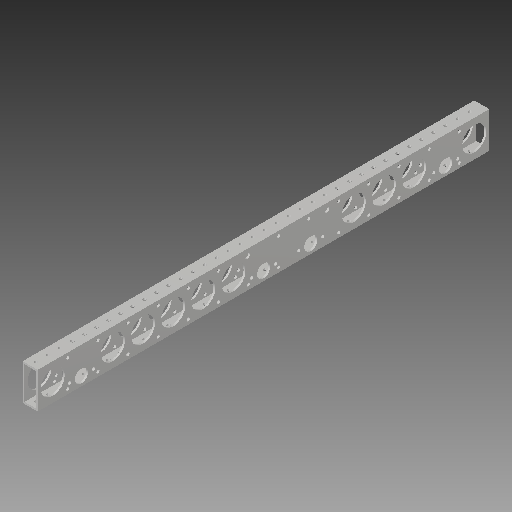
# Autodesk Inventor part: Side Extrusion
Saved by Autodesk Inventor 2019.4 (Build 234330000, 330)
## iProperties
Created: 2019-12-11
Part Number: Side Extrusion
Material: Aluminum 6061
Document SubType Name: Modeling
Designer: Mark
Mass: 702.477 g
Surface Area: 1912.79 cm^2
Volume: 260.177 cm^3
Density: 2.7 g/cm^3
Appearance: Aluminum - Flat
Author: Mark
Autodesk Inventor part; units mm, degrees
ref_plane "YZ Plane" through (0, 0, 0) normal (1, 0, 0) x (0, 1, 0)
ref_plane "XZ Plane" through (0, 0, 0) normal (0, 1, 0) x (-1, 0, 0)
ref_plane "XY Plane" through (0, 0, 0) normal (0, 0, 1) x (1, 0, 0)
sketch "Sketch1" plane through (0, 0, 0) normal (0, 0, 1) x (1, 0, 0)
  line L0 (-12.5, -30) -> (12.5, -30)
  line L1 (12.5, -30) -> (12.5, 30)
  line L2 (12.5, 30) -> (-12.5, 30)
  line L3 (-12.5, 30) -> (-12.5, -30)
  line L4 (-12.5, -30) -> (12.5, 30) construction
  line L5 (12.5, -30) -> (-12.5, 30) construction
  line L6 (-9.5, -27) -> (9.5, -27)
  line L7 (9.5, -27) -> (9.5, 27)
  line L8 (9.5, 27) -> (-9.5, 27)
  line L9 (-9.5, 27) -> (-9.5, -27)
  line L10 (-9.5, -27) -> (9.5, 27) construction
  line L11 (9.5, -27) -> (-9.5, 27) construction
  point P0 (0, 0)
  dimension "d0" = 25
  dimension "d1" = 60
  dimension "d2" = 19
  dimension "d3" = 54
  constraints: 24 end point, 4 midpoint, 4 parallel, 2 horizontal, 2 perpendicular
  measures "d0" distance of L2.end L1.end
  measures "d1" distance of L1.end L0.end
  measures "d2" distance of L8.end L7.end
  measures "d3" distance of L7.end L6.end
extrude "Extrusion1" add sketch "Sketch1" along normal blind 750
sketch "Sketch2" plane through (12.5, -30, 0) normal (1, 0, 0) x (0, 0, -1)
  circle A0 centre (-375, 15) radius 11
  circle A1 centre (-677.46, 15) radius 11
  circle A2 centre (-72.54, 15) radius 11
  line L0 (0, 60) -> (-750, 60) projected
  line L1 (-750, 0) -> (-750, 60) projected
  circle A3 centre (-677.46, 15) radius 20 construction
  circle A4 centre (-697.46, 15) radius 2.75
  circle A5 centre (-657.46, 15) radius 2.75
  line L2 (-677.46, 15) -> (-697.46, 15) construction
  line L3 (-677.46, 15) -> (-657.46, 15) construction
  line L4 (-375, 15) -> (-375, 60)
  circle A6 centre (-395, 15) radius 2.75
  line L5 (0, 0) -> (-750, 0) projected
  circle A7 centre (-52.54, 15) radius 2.75
  circle A8 centre (-92.54, 15) radius 2.75
  circle A9 centre (-355, 15) radius 2.75
  circle A10 centre (-316.54, 15) radius 2.75
  circle A11 centre (-276.54, 15) radius 2.75
  circle A12 centre (-296.54, 15) radius 11
  point P0 (0, 30)
  dimension "d6" = 22
  dimension "d7" = 22
  dimension "d8" = 22
  dimension "d9" = 45
  dimension "d10" = 45
  dimension "d11" = 45
  dimension "d12" = 375
  dimension "d13" = 302.46
  dimension "d14" = 302.46
  dimension "d33" = 40
  dimension "d34" = 5.5
  dimension "d35" = 5.5
  dimension "d36" = 40
  dimension "d37" = 180
  dimension "d38" = 5.5
  dimension "d39" = 20
  dimension "d41" = 45
  dimension "d44" = 78.46
  constraints: 13 centre point, 6 end point, 3 horizontal, 3 symmetric about line, 2 point on circle, 1 coincident, 1 collinear, 1 midpoint, 9 other
  measures "d6" diameter of A0
  measures "d7" diameter of A1
  measures "d8" diameter of A2
  measures "d9" distance from line of L0 L4.start
  measures "d10" distance from line of L0 A2.centre
  measures "d11" distance from line of L0 A1.centre
  measures "d12" distance from line of L1 L4.start
  measures "d13" distance of L4.start A1.centre
  measures "d14" distance of L4.start A2.centre
  measures "d33" diameter of A3
  measures "d34" diameter of A4
  measures "d35" diameter of A5
  measures "d36" distance of A5.centre L2.end
  measures "d37" angle of L2 L3
  measures "d38" diameter of A6
  measures "d39" distance of L4.start A6.centre
  measures "d41" distance from line of L0 A6.centre
  measures "d44" distance of A6.centre A10.centre
extrude "Extrusion2" cut sketch "Sketch2" against normal through all
sketch "Sketch4" plane through (-12.5, 30, 0) normal (0, 1, 0) x (1, 0, 0)
  circle A0 centre (12.5, -20) radius 2.75
  line L0 (25, 0) -> (25, -750) projected
  line L1 (25, 0) -> (0, 0) projected
  circle A1 centre (12.5, -40) radius 2.75
  circle A2 centre (12.5, -60) radius 2.75
  circle A3 centre (12.5, -80) radius 2.75
  circle A4 centre (12.5, -100) radius 2.75
  circle A5 centre (12.5, -120) radius 2.75
  circle A6 centre (12.5, -140) radius 2.75
  circle A7 centre (12.5, -160) radius 2.75
  circle A8 centre (12.5, -180) radius 2.75
  circle A9 centre (12.5, -200) radius 2.75
  circle A10 centre (12.5, -220) radius 2.75
  circle A11 centre (12.5, -240) radius 2.75
  circle A12 centre (12.5, -260) radius 2.75
  circle A13 centre (12.5, -280) radius 2.75
  circle A14 centre (12.5, -300) radius 2.75
  circle A15 centre (12.5, -320) radius 2.75
  circle A16 centre (12.5, -340) radius 2.75
  circle A17 centre (12.5, -360) radius 2.75
  circle A18 centre (12.5, -380) radius 2.75
  circle A19 centre (12.5, -400) radius 2.75
  circle A20 centre (12.5, -420) radius 2.75
  circle A21 centre (12.5, -440) radius 2.75
  circle A22 centre (12.5, -460) radius 2.75
  circle A23 centre (12.5, -480) radius 2.75
  circle A24 centre (12.5, -500) radius 2.75
  circle A25 centre (12.5, -520) radius 2.75
  circle A26 centre (12.5, -540) radius 2.75
  circle A27 centre (12.5, -560) radius 2.75
  circle A28 centre (12.5, -580) radius 2.75
  circle A29 centre (12.5, -600) radius 2.75
  circle A30 centre (12.5, -620) radius 2.75
  circle A31 centre (12.5, -640) radius 2.75
  circle A32 centre (12.5, -660) radius 2.75
  circle A33 centre (12.5, -680) radius 2.75
  circle A34 centre (12.5, -700) radius 2.75
  circle A35 centre (12.5, -720) radius 2.75
  circle A36 centre (12.5, -740) radius 2.75
  circle A37 centre (12.5, -760) radius 2.75
  circle A38 centre (12.5, -780) radius 2.75
  circle A39 centre (12.5, -800) radius 2.75
  point P0 (12.5, 0)
  dimension "d21" = 5.5
  dimension "d22" = 12.5
  dimension "d23" = 20
  dimension "d26" = 20
  constraints: 40 centre point, 1 vertical, 78 other
  measures "d21" diameter of A0
  measures "d22" distance from line of L0 A0.centre
  measures "d23" distance from line of L1 A0.centre
  measures "d26" distance of A0.centre A1.centre
extrude "Extrusion3" cut sketch "Sketch4" against normal blind 100 contours A0 | A1 | A2 | A3 | A4 | A5 | A6 | A7 | A8 | A9 | A10 | A11 | A12 | A13 | A14 | A15 | A16 | A17 | A18 | A19 | A20 | A21 | A22 | A23 | A24 | A25 | A26 | A27 | A28 | A29 | A30 | A31 | A32 | A33 | A34 | A35 | A36 | A37 | A38
sketch "Sketch5" plane through (12.5, -30, 0) normal (1, 0, 0) x (0, 0, -1)
  circle A0 centre (-401.79, 50) radius 4.25
  line L0 (0, 60) -> (-750, 60) projected
  line L1 (-750, 0) -> (-750, 60) projected
  circle A1 centre (-269.75, 50) radius 4.25
  point P0 (0, 30)
  dimension "d49" = 8.5
  dimension "d50" = 10
  dimension "d51" = 348.21
  dimension "d52" = 8.5
  dimension "d53" = 10
  dimension "d54" = 132.04
  constraints: 2 centre point
  measures "d49" diameter of A0
  measures "d50" distance from line of L0 A0.centre
  measures "d51" distance from line of L1 A0.centre
  measures "d52" diameter of A1
  measures "d53" distance from line of L0 A1.centre
  measures "d54" distance of A0.centre A1.centre
extrude "Extrusion4" cut sketch "Sketch5" against normal blind 50
sketch "Sketch6" plane through (12.5, -30, 0) normal (1, 0, 0) x (0, 0, -1)
  line L0 (0, 60) -> (-750, 60) projected
  line L1 (-375, 60) -> (-375, 0) construction
  line L2 (-375, 60) -> (-315, 60) construction
  circle A0 centre (-375, 30) radius 20
  line L3 (-400, 7.5) -> (-350, 7.5) construction
  line L4 (-350, 7.5) -> (-350, 52.5) construction
  line L5 (-350, 52.5) -> (-400, 52.5) construction
  line L6 (-400, 52.5) -> (-400, 7.5) construction
  line L7 (-400, 7.5) -> (-350, 52.5) construction
  line L8 (-350, 7.5) -> (-400, 52.5) construction
  circle A1 centre (-350, 52.5) radius 2.75
  circle A2 centre (-400, 52.5) radius 2.75
  circle A3 centre (-400, 7.5) radius 2.75
  circle A4 centre (-350, 7.5) radius 2.75
  circle A5 centre (-450, 52.5) radius 2.75
  circle A6 centre (-450, 7.5) radius 2.75
  circle A7 centre (-400, 7.5) radius 2.75
  circle A8 centre (-425, 30) radius 20
  circle A9 centre (-400, 52.5) radius 2.75
  circle A10 centre (-500, 52.5) radius 2.75
  circle A11 centre (-500, 7.5) radius 2.75
  circle A12 centre (-450, 7.5) radius 2.75
  circle A13 centre (-475, 30) radius 20
  circle A14 centre (-450, 52.5) radius 2.75
  circle A15 centre (-550, 52.5) radius 2.75
  circle A16 centre (-550, 7.5) radius 2.75
  circle A17 centre (-500, 7.5) radius 2.75
  circle A18 centre (-525, 30) radius 20
  circle A19 centre (-500, 52.5) radius 2.75
  circle A20 centre (-600, 52.5) radius 2.75
  circle A21 centre (-600, 7.5) radius 2.75
  circle A22 centre (-550, 7.5) radius 2.75
  circle A23 centre (-575, 30) radius 20
  circle A24 centre (-550, 52.5) radius 2.75
  circle A25 centre (-650, 52.5) radius 2.75
  circle A26 centre (-650, 7.5) radius 2.75
  circle A27 centre (-600, 7.5) radius 2.75
  circle A28 centre (-625, 30) radius 20
  circle A29 centre (-600, 52.5) radius 2.75
  circle A30 centre (-700, 52.5) radius 2.75
  circle A31 centre (-700, 7.5) radius 2.75
  circle A32 centre (-650, 7.5) radius 2.75
  circle A33 centre (-675, 30) radius 20
  circle A34 centre (-650, 52.5) radius 2.75
  circle A35 centre (-750, 52.5) radius 2.75
  circle A36 centre (-750, 7.5) radius 2.75
  circle A37 centre (-700, 7.5) radius 2.75
  circle A38 centre (-725, 30) radius 20
  circle A39 centre (-700, 52.5) radius 2.75
  circle A40 centre (-800, 52.5) radius 2.75
  circle A41 centre (-800, 7.5) radius 2.75
  circle A42 centre (-750, 7.5) radius 2.75
  circle A43 centre (-775, 30) radius 20
  circle A44 centre (-750, 52.5) radius 2.75
  circle A45 centre (-850, 52.5) radius 2.75
  circle A46 centre (-850, 7.5) radius 2.75
  circle A47 centre (-800, 7.5) radius 2.75
  circle A48 centre (-825, 30) radius 20
  circle A49 centre (-800, 52.5) radius 2.75
  circle A50 centre (-350, 52.5) radius 2.75
  circle A51 centre (-350, 7.5) radius 2.75
  circle A52 centre (-300, 7.5) radius 2.75
  circle A53 centre (-325, 30) radius 20
  circle A54 centre (-300, 52.5) radius 2.75
  circle A55 centre (-400, 52.5) radius 2.75
  circle A56 centre (-400, 7.5) radius 2.75
  circle A57 centre (-350, 7.5) radius 2.75
  circle A58 centre (-375, 30) radius 20
  circle A59 centre (-350, 52.5) radius 2.75
  circle A60 centre (-450, 52.5) radius 2.75
  circle A61 centre (-450, 7.5) radius 2.75
  circle A62 centre (-400, 7.5) radius 2.75
  circle A63 centre (-425, 30) radius 20
  circle A64 centre (-400, 52.5) radius 2.75
  circle A65 centre (-500, 52.5) radius 2.75
  circle A66 centre (-500, 7.5) radius 2.75
  circle A67 centre (-450, 7.5) radius 2.75
  circle A68 centre (-475, 30) radius 20
  circle A69 centre (-450, 52.5) radius 2.75
  circle A70 centre (-550, 52.5) radius 2.75
  circle A71 centre (-550, 7.5) radius 2.75
  circle A72 centre (-500, 7.5) radius 2.75
  circle A73 centre (-525, 30) radius 20
  circle A74 centre (-500, 52.5) radius 2.75
  circle A75 centre (-600, 52.5) radius 2.75
  circle A76 centre (-600, 7.5) radius 2.75
  circle A77 centre (-550, 7.5) radius 2.75
  circle A78 centre (-575, 30) radius 20
  circle A79 centre (-550, 52.5) radius 2.75
  circle A80 centre (-650, 52.5) radius 2.75
  circle A81 centre (-650, 7.5) radius 2.75
  circle A82 centre (-600, 7.5) radius 2.75
  circle A83 centre (-625, 30) radius 20
  circle A84 centre (-600, 52.5) radius 2.75
  circle A85 centre (-700, 52.5) radius 2.75
  circle A86 centre (-700, 7.5) radius 2.75
  circle A87 centre (-650, 7.5) radius 2.75
  circle A88 centre (-675, 30) radius 20
  circle A89 centre (-650, 52.5) radius 2.75
  circle A90 centre (-750, 52.5) radius 2.75
  circle A91 centre (-750, 7.5) radius 2.75
  circle A92 centre (-700, 7.5) radius 2.75
  circle A93 centre (-725, 30) radius 20
  circle A94 centre (-700, 52.5) radius 2.75
  circle A95 centre (-800, 52.5) radius 2.75
  circle A96 centre (-800, 7.5) radius 2.75
  circle A97 centre (-750, 7.5) radius 2.75
  circle A98 centre (-775, 30) radius 20
  circle A99 centre (-750, 52.5) radius 2.75
  circle A100 centre (-300, 52.5) radius 2.75
  circle A101 centre (-300, 7.5) radius 2.75
  circle A102 centre (-250, 7.5) radius 2.75
  circle A103 centre (-275, 30) radius 20
  circle A104 centre (-250, 52.5) radius 2.75
  circle A105 centre (-350, 52.5) radius 2.75
  circle A106 centre (-350, 7.5) radius 2.75
  circle A107 centre (-300, 7.5) radius 2.75
  circle A108 centre (-325, 30) radius 20
  circle A109 centre (-300, 52.5) radius 2.75
  circle A110 centre (-400, 52.5) radius 2.75
  circle A111 centre (-400, 7.5) radius 2.75
  circle A112 centre (-350, 7.5) radius 2.75
  circle A113 centre (-375, 30) radius 20
  circle A114 centre (-350, 52.5) radius 2.75
  circle A115 centre (-450, 52.5) radius 2.75
  circle A116 centre (-450, 7.5) radius 2.75
  circle A117 centre (-400, 7.5) radius 2.75
  circle A118 centre (-425, 30) radius 20
  circle A119 centre (-400, 52.5) radius 2.75
  circle A120 centre (-500, 52.5) radius 2.75
  circle A121 centre (-500, 7.5) radius 2.75
  circle A122 centre (-450, 7.5) radius 2.75
  circle A123 centre (-475, 30) radius 20
  circle A124 centre (-450, 52.5) radius 2.75
  circle A125 centre (-550, 52.5) radius 2.75
  circle A126 centre (-550, 7.5) radius 2.75
  circle A127 centre (-500, 7.5) radius 2.75
  circle A128 centre (-525, 30) radius 20
  circle A129 centre (-500, 52.5) radius 2.75
  circle A130 centre (-600, 52.5) radius 2.75
  circle A131 centre (-600, 7.5) radius 2.75
  circle A132 centre (-550, 7.5) radius 2.75
  circle A133 centre (-575, 30) radius 20
  circle A134 centre (-550, 52.5) radius 2.75
  circle A135 centre (-650, 52.5) radius 2.75
  circle A136 centre (-650, 7.5) radius 2.75
  circle A137 centre (-600, 7.5) radius 2.75
  circle A138 centre (-625, 30) radius 20
  circle A139 centre (-600, 52.5) radius 2.75
  circle A140 centre (-700, 52.5) radius 2.75
  circle A141 centre (-700, 7.5) radius 2.75
  circle A142 centre (-650, 7.5) radius 2.75
  circle A143 centre (-675, 30) radius 20
  circle A144 centre (-650, 52.5) radius 2.75
  circle A145 centre (-750, 52.5) radius 2.75
  circle A146 centre (-750, 7.5) radius 2.75
  circle A147 centre (-700, 7.5) radius 2.75
  circle A148 centre (-725, 30) radius 20
  circle A149 centre (-700, 52.5) radius 2.75
  circle A150 centre (-250, 52.5) radius 2.75
  circle A151 centre (-250, 7.5) radius 2.75
  circle A152 centre (-200, 7.5) radius 2.75
  circle A153 centre (-225, 30) radius 20
  circle A154 centre (-200, 52.5) radius 2.75
  circle A155 centre (-300, 52.5) radius 2.75
  circle A156 centre (-300, 7.5) radius 2.75
  circle A157 centre (-250, 7.5) radius 2.75
  circle A158 centre (-275, 30) radius 20
  circle A159 centre (-250, 52.5) radius 2.75
  circle A160 centre (-350, 52.5) radius 2.75
  circle A161 centre (-350, 7.5) radius 2.75
  circle A162 centre (-300, 7.5) radius 2.75
  circle A163 centre (-325, 30) radius 20
  circle A164 centre (-300, 52.5) radius 2.75
  circle A165 centre (-400, 52.5) radius 2.75
  circle A166 centre (-400, 7.5) radius 2.75
  circle A167 centre (-350, 7.5) radius 2.75
  circle A168 centre (-375, 30) radius 20
  circle A169 centre (-350, 52.5) radius 2.75
  circle A170 centre (-450, 52.5) radius 2.75
  circle A171 centre (-450, 7.5) radius 2.75
  circle A172 centre (-400, 7.5) radius 2.75
  circle A173 centre (-425, 30) radius 20
  circle A174 centre (-400, 52.5) radius 2.75
  circle A175 centre (-500, 52.5) radius 2.75
  circle A176 centre (-500, 7.5) radius 2.75
  circle A177 centre (-450, 7.5) radius 2.75
  circle A178 centre (-475, 30) radius 20
  circle A179 centre (-450, 52.5) radius 2.75
  circle A180 centre (-550, 52.5) radius 2.75
  circle A181 centre (-550, 7.5) radius 2.75
  circle A182 centre (-500, 7.5) radius 2.75
  circle A183 centre (-525, 30) radius 20
  circle A184 centre (-500, 52.5) radius 2.75
  circle A185 centre (-600, 52.5) radius 2.75
  circle A186 centre (-600, 7.5) radius 2.75
  circle A187 centre (-550, 7.5) radius 2.75
  circle A188 centre (-575, 30) radius 20
  circle A189 centre (-550, 52.5) radius 2.75
  circle A190 centre (-650, 52.5) radius 2.75
  circle A191 centre (-650, 7.5) radius 2.75
  circle A192 centre (-600, 7.5) radius 2.75
  circle A193 centre (-625, 30) radius 20
  circle A194 centre (-600, 52.5) radius 2.75
  circle A195 centre (-700, 52.5) radius 2.75
  circle A196 centre (-700, 7.5) radius 2.75
  circle A197 centre (-650, 7.5) radius 2.75
  circle A198 centre (-675, 30) radius 20
  circle A199 centre (-650, 52.5) radius 2.75
  circle A200 centre (-200, 52.5) radius 2.75
  circle A201 centre (-200, 7.5) radius 2.75
  circle A202 centre (-150, 7.5) radius 2.75
  circle A203 centre (-175, 30) radius 20
  circle A204 centre (-150, 52.5) radius 2.75
  circle A205 centre (-250, 52.5) radius 2.75
  circle A206 centre (-250, 7.5) radius 2.75
  circle A207 centre (-200, 7.5) radius 2.75
  circle A208 centre (-225, 30) radius 20
  circle A209 centre (-200, 52.5) radius 2.75
  circle A210 centre (-300, 52.5) radius 2.75
  circle A211 centre (-300, 7.5) radius 2.75
  circle A212 centre (-250, 7.5) radius 2.75
  circle A213 centre (-275, 30) radius 20
  circle A214 centre (-250, 52.5) radius 2.75
  circle A215 centre (-350, 52.5) radius 2.75
  circle A216 centre (-350, 7.5) radius 2.75
  circle A217 centre (-300, 7.5) radius 2.75
  circle A218 centre (-325, 30) radius 20
  circle A219 centre (-300, 52.5) radius 2.75
  circle A220 centre (-400, 52.5) radius 2.75
  circle A221 centre (-400, 7.5) radius 2.75
  circle A222 centre (-350, 7.5) radius 2.75
  circle A223 centre (-375, 30) radius 20
  circle A224 centre (-350, 52.5) radius 2.75
  circle A225 centre (-450, 52.5) radius 2.75
  circle A226 centre (-450, 7.5) radius 2.75
  circle A227 centre (-400, 7.5) radius 2.75
  circle A228 centre (-425, 30) radius 20
  circle A229 centre (-400, 52.5) radius 2.75
  circle A230 centre (-500, 52.5) radius 2.75
  circle A231 centre (-500, 7.5) radius 2.75
  circle A232 centre (-450, 7.5) radius 2.75
  circle A233 centre (-475, 30) radius 20
  circle A234 centre (-450, 52.5) radius 2.75
  circle A235 centre (-550, 52.5) radius 2.75
  circle A236 centre (-550, 7.5) radius 2.75
  circle A237 centre (-500, 7.5) radius 2.75
  circle A238 centre (-525, 30) radius 20
  circle A239 centre (-500, 52.5) radius 2.75
  circle A240 centre (-600, 52.5) radius 2.75
  circle A241 centre (-600, 7.5) radius 2.75
  circle A242 centre (-550, 7.5) radius 2.75
  circle A243 centre (-575, 30) radius 20
  circle A244 centre (-550, 52.5) radius 2.75
  circle A245 centre (-650, 52.5) radius 2.75
  circle A246 centre (-650, 7.5) radius 2.75
  circle A247 centre (-600, 7.5) radius 2.75
  circle A248 centre (-625, 30) radius 20
  circle A249 centre (-600, 52.5) radius 2.75
  circle A250 centre (-150, 52.5) radius 2.75
  circle A251 centre (-150, 7.5) radius 2.75
  circle A252 centre (-100, 7.5) radius 2.75
  circle A253 centre (-125, 30) radius 20
  circle A254 centre (-100, 52.5) radius 2.75
  circle A255 centre (-200, 52.5) radius 2.75
  circle A256 centre (-200, 7.5) radius 2.75
  circle A257 centre (-150, 7.5) radius 2.75
  circle A258 centre (-175, 30) radius 20
  circle A259 centre (-150, 52.5) radius 2.75
  circle A260 centre (-250, 52.5) radius 2.75
  circle A261 centre (-250, 7.5) radius 2.75
  circle A262 centre (-200, 7.5) radius 2.75
  circle A263 centre (-225, 30) radius 20
  circle A264 centre (-200, 52.5) radius 2.75
  circle A265 centre (-300, 52.5) radius 2.75
  circle A266 centre (-300, 7.5) radius 2.75
  circle A267 centre (-250, 7.5) radius 2.75
  circle A268 centre (-275, 30) radius 20
  circle A269 centre (-250, 52.5) radius 2.75
  circle A270 centre (-350, 52.5) radius 2.75
  circle A271 centre (-350, 7.5) radius 2.75
  circle A272 centre (-300, 7.5) radius 2.75
  circle A273 centre (-325, 30) radius 20
  circle A274 centre (-300, 52.5) radius 2.75
  circle A275 centre (-400, 52.5) radius 2.75
  circle A276 centre (-400, 7.5) radius 2.75
  circle A277 centre (-350, 7.5) radius 2.75
  circle A278 centre (-375, 30) radius 20
  circle A279 centre (-350, 52.5) radius 2.75
  circle A280 centre (-450, 52.5) radius 2.75
  circle A281 centre (-450, 7.5) radius 2.75
  circle A282 centre (-400, 7.5) radius 2.75
  circle A283 centre (-425, 30) radius 20
  circle A284 centre (-400, 52.5) radius 2.75
  circle A285 centre (-500, 52.5) radius 2.75
  circle A286 centre (-500, 7.5) radius 2.75
  circle A287 centre (-450, 7.5) radius 2.75
  circle A288 centre (-475, 30) radius 20
  circle A289 centre (-450, 52.5) radius 2.75
  circle A290 centre (-550, 52.5) radius 2.75
  circle A291 centre (-550, 7.5) radius 2.75
  circle A292 centre (-500, 7.5) radius 2.75
  circle A293 centre (-525, 30) radius 20
  circle A294 centre (-500, 52.5) radius 2.75
  circle A295 centre (-600, 52.5) radius 2.75
  circle A296 centre (-600, 7.5) radius 2.75
  circle A297 centre (-550, 7.5) radius 2.75
  circle A298 centre (-575, 30) radius 20
  circle A299 centre (-550, 52.5) radius 2.75
  circle A300 centre (-100, 52.5) radius 2.75
  circle A301 centre (-100, 7.5) radius 2.75
  circle A302 centre (-50, 7.5) radius 2.75
  circle A303 centre (-75, 30) radius 20
  circle A304 centre (-50, 52.5) radius 2.75
  circle A305 centre (-150, 52.5) radius 2.75
  circle A306 centre (-150, 7.5) radius 2.75
  circle A307 centre (-100, 7.5) radius 2.75
  circle A308 centre (-125, 30) radius 20
  circle A309 centre (-100, 52.5) radius 2.75
  circle A310 centre (-200, 52.5) radius 2.75
  circle A311 centre (-200, 7.5) radius 2.75
  circle A312 centre (-150, 7.5) radius 2.75
  circle A313 centre (-175, 30) radius 20
  circle A314 centre (-150, 52.5) radius 2.75
  circle A315 centre (-250, 52.5) radius 2.75
  circle A316 centre (-250, 7.5) radius 2.75
  circle A317 centre (-200, 7.5) radius 2.75
  circle A318 centre (-225, 30) radius 20
  circle A319 centre (-200, 52.5) radius 2.75
  circle A320 centre (-300, 52.5) radius 2.75
  circle A321 centre (-300, 7.5) radius 2.75
  circle A322 centre (-250, 7.5) radius 2.75
  circle A323 centre (-275, 30) radius 20
  circle A324 centre (-250, 52.5) radius 2.75
  circle A325 centre (-350, 52.5) radius 2.75
  circle A326 centre (-350, 7.5) radius 2.75
  circle A327 centre (-300, 7.5) radius 2.75
  circle A328 centre (-325, 30) radius 20
  circle A329 centre (-300, 52.5) radius 2.75
  circle A330 centre (-400, 52.5) radius 2.75
  circle A331 centre (-400, 7.5) radius 2.75
  circle A332 centre (-350, 7.5) radius 2.75
  circle A333 centre (-375, 30) radius 20
  circle A334 centre (-350, 52.5) radius 2.75
  circle A335 centre (-450, 52.5) radius 2.75
  circle A336 centre (-450, 7.5) radius 2.75
  circle A337 centre (-400, 7.5) radius 2.75
  circle A338 centre (-425, 30) radius 20
  circle A339 centre (-400, 52.5) radius 2.75
  circle A340 centre (-500, 52.5) radius 2.75
  circle A341 centre (-500, 7.5) radius 2.75
  circle A342 centre (-450, 7.5) radius 2.75
  circle A343 centre (-475, 30) radius 20
  circle A344 centre (-450, 52.5) radius 2.75
  circle A345 centre (-550, 52.5) radius 2.75
  circle A346 centre (-550, 7.5) radius 2.75
  circle A347 centre (-500, 7.5) radius 2.75
  circle A348 centre (-525, 30) radius 20
  circle A349 centre (-500, 52.5) radius 2.75
  circle A350 centre (-50, 52.5) radius 2.75
  circle A351 centre (-50, 7.5) radius 2.75
  circle A352 centre (0, 7.5) radius 2.75
  circle A353 centre (-25, 30) radius 20
  circle A354 centre (0, 52.5) radius 2.75
  circle A355 centre (-100, 52.5) radius 2.75
  circle A356 centre (-100, 7.5) radius 2.75
  circle A357 centre (-50, 7.5) radius 2.75
  circle A358 centre (-75, 30) radius 20
  circle A359 centre (-50, 52.5) radius 2.75
  circle A360 centre (-150, 52.5) radius 2.75
  circle A361 centre (-150, 7.5) radius 2.75
  circle A362 centre (-100, 7.5) radius 2.75
  circle A363 centre (-125, 30) radius 20
  circle A364 centre (-100, 52.5) radius 2.75
  circle A365 centre (-200, 52.5) radius 2.75
  circle A366 centre (-200, 7.5) radius 2.75
  circle A367 centre (-150, 7.5) radius 2.75
  circle A368 centre (-175, 30) radius 20
  circle A369 centre (-150, 52.5) radius 2.75
  circle A370 centre (-250, 52.5) radius 2.75
  circle A371 centre (-250, 7.5) radius 2.75
  circle A372 centre (-200, 7.5) radius 2.75
  circle A373 centre (-225, 30) radius 20
  circle A374 centre (-200, 52.5) radius 2.75
  circle A375 centre (-300, 52.5) radius 2.75
  circle A376 centre (-300, 7.5) radius 2.75
  circle A377 centre (-250, 7.5) radius 2.75
  circle A378 centre (-275, 30) radius 20
  circle A379 centre (-250, 52.5) radius 2.75
  circle A380 centre (-350, 52.5) radius 2.75
  circle A381 centre (-350, 7.5) radius 2.75
  circle A382 centre (-300, 7.5) radius 2.75
  circle A383 centre (-325, 30) radius 20
  circle A384 centre (-300, 52.5) radius 2.75
  circle A385 centre (-400, 52.5) radius 2.75
  circle A386 centre (-400, 7.5) radius 2.75
  circle A387 centre (-350, 7.5) radius 2.75
  circle A388 centre (-375, 30) radius 20
  circle A389 centre (-350, 52.5) radius 2.75
  circle A390 centre (-450, 52.5) radius 2.75
  circle A391 centre (-450, 7.5) radius 2.75
  circle A392 centre (-400, 7.5) radius 2.75
  circle A393 centre (-425, 30) radius 20
  circle A394 centre (-400, 52.5) radius 2.75
  circle A395 centre (-500, 52.5) radius 2.75
  circle A396 centre (-500, 7.5) radius 2.75
  circle A397 centre (-450, 7.5) radius 2.75
  circle A398 centre (-475, 30) radius 20
  circle A399 centre (-450, 52.5) radius 2.75
  circle A400 centre (0, 52.5) radius 2.75
  circle A401 centre (0, 7.5) radius 2.75
  circle A402 centre (50, 7.5) radius 2.75
  circle A403 centre (25, 30) radius 20
  circle A404 centre (50, 52.5) radius 2.75
  circle A405 centre (-50, 52.5) radius 2.75
  circle A406 centre (-50, 7.5) radius 2.75
  circle A407 centre (0, 7.5) radius 2.75
  circle A408 centre (-25, 30) radius 20
  circle A409 centre (0, 52.5) radius 2.75
  circle A410 centre (-100, 52.5) radius 2.75
  circle A411 centre (-100, 7.5) radius 2.75
  circle A412 centre (-50, 7.5) radius 2.75
  circle A413 centre (-75, 30) radius 20
  circle A414 centre (-50, 52.5) radius 2.75
  circle A415 centre (-150, 52.5) radius 2.75
  circle A416 centre (-150, 7.5) radius 2.75
  circle A417 centre (-100, 7.5) radius 2.75
  circle A418 centre (-125, 30) radius 20
  circle A419 centre (-100, 52.5) radius 2.75
  circle A420 centre (-200, 52.5) radius 2.75
  circle A421 centre (-200, 7.5) radius 2.75
  circle A422 centre (-150, 7.5) radius 2.75
  circle A423 centre (-175, 30) radius 20
  circle A424 centre (-150, 52.5) radius 2.75
  circle A425 centre (-250, 52.5) radius 2.75
  circle A426 centre (-250, 7.5) radius 2.75
  circle A427 centre (-200, 7.5) radius 2.75
  circle A428 centre (-225, 30) radius 20
  circle A429 centre (-200, 52.5) radius 2.75
  circle A430 centre (-300, 52.5) radius 2.75
  circle A431 centre (-300, 7.5) radius 2.75
  circle A432 centre (-250, 7.5) radius 2.75
  circle A433 centre (-275, 30) radius 20
  circle A434 centre (-250, 52.5) radius 2.75
  circle A435 centre (-350, 52.5) radius 2.75
  circle A436 centre (-350, 7.5) radius 2.75
  circle A437 centre (-300, 7.5) radius 2.75
  circle A438 centre (-325, 30) radius 20
  circle A439 centre (-300, 52.5) radius 2.75
  circle A440 centre (-400, 52.5) radius 2.75
  circle A441 centre (-400, 7.5) radius 2.75
  circle A442 centre (-350, 7.5) radius 2.75
  circle A443 centre (-375, 30) radius 20
  circle A444 centre (-350, 52.5) radius 2.75
  circle A445 centre (-450, 52.5) radius 2.75
  circle A446 centre (-450, 7.5) radius 2.75
  circle A447 centre (-400, 7.5) radius 2.75
  circle A448 centre (-425, 30) radius 20
  circle A449 centre (-400, 52.5) radius 2.75
  circle A450 centre (50, 52.5) radius 2.75
  circle A451 centre (50, 7.5) radius 2.75
  circle A452 centre (100, 7.5) radius 2.75
  circle A453 centre (75, 30) radius 20
  circle A454 centre (100, 52.5) radius 2.75
  circle A455 centre (0, 52.5) radius 2.75
  circle A456 centre (0, 7.5) radius 2.75
  circle A457 centre (50, 7.5) radius 2.75
  circle A458 centre (25, 30) radius 20
  circle A459 centre (50, 52.5) radius 2.75
  circle A460 centre (-50, 52.5) radius 2.75
  circle A461 centre (-50, 7.5) radius 2.75
  circle A462 centre (0, 7.5) radius 2.75
  circle A463 centre (-25, 30) radius 20
  circle A464 centre (0, 52.5) radius 2.75
  circle A465 centre (-100, 52.5) radius 2.75
  circle A466 centre (-100, 7.5) radius 2.75
  circle A467 centre (-50, 7.5) radius 2.75
  circle A468 centre (-75, 30) radius 20
  circle A469 centre (-50, 52.5) radius 2.75
  circle A470 centre (-150, 52.5) radius 2.75
  circle A471 centre (-150, 7.5) radius 2.75
  circle A472 centre (-100, 7.5) radius 2.75
  circle A473 centre (-125, 30) radius 20
  circle A474 centre (-100, 52.5) radius 2.75
  circle A475 centre (-200, 52.5) radius 2.75
  circle A476 centre (-200, 7.5) radius 2.75
  circle A477 centre (-150, 7.5) radius 2.75
  circle A478 centre (-175, 30) radius 20
  circle A479 centre (-150, 52.5) radius 2.75
  circle A480 centre (-250, 52.5) radius 2.75
  circle A481 centre (-250, 7.5) radius 2.75
  circle A482 centre (-200, 7.5) radius 2.75
  circle A483 centre (-225, 30) radius 20
  circle A484 centre (-200, 52.5) radius 2.75
  circle A485 centre (-300, 52.5) radius 2.75
  circle A486 centre (-300, 7.5) radius 2.75
  circle A487 centre (-250, 7.5) radius 2.75
  circle A488 centre (-275, 30) radius 20
  circle A489 centre (-250, 52.5) radius 2.75
  circle A490 centre (-350, 52.5) radius 2.75
  circle A491 centre (-350, 7.5) radius 2.75
  circle A492 centre (-300, 7.5) radius 2.75
  circle A493 centre (-325, 30) radius 20
  circle A494 centre (-300, 52.5) radius 2.75
  circle A495 centre (-400, 52.5) radius 2.75
  circle A496 centre (-400, 7.5) radius 2.75
  circle A497 centre (-350, 7.5) radius 2.75
  circle A498 centre (-375, 30) radius 20
  circle A499 centre (-350, 52.5) radius 2.75
  point P0 (0, 30)
  dimension "d57" = 60
  dimension "d58" = 90
  dimension "d59" = 40
  dimension "d60" = 50
  dimension "d61" = 45
  dimension "d62" = 5.5
  dimension "d63" = 5.5
  dimension "d64" = 5.5
  dimension "d65" = 5.5
  dimension "d68" = 50
  dimension "d71" = 50
  constraints: 500 centre point, 16 end point, 4 coincident, 4 horizontal, 4 midpoint, 2 parallel, 2 perpendicular, 1 vertical, 990 other
  measures "d57" distance of L1.start L1.end
  measures "d58" angle of L1 L2
  measures "d59" diameter of A0
  measures "d60" distance of L5.end L4.end
  measures "d61" distance of L4.end L3.end
  measures "d62" diameter of A1
  measures "d63" diameter of A2
  measures "d64" diameter of A3
  measures "d65" diameter of A4
  measures "d68" distance of A2.centre A5.centre
  measures "d71" distance of A2.centre A50.centre
extrude "Extrusion5" cut sketch "Sketch6" against normal blind 50 contours A1 | A3 | A4 | A5 | A6 | A8 | A10 | A11 | A13 | A15 | A16 | A18 | A20 | A21 | A23 | A25 | A26 | A28 | A30 | A31 | A38 | A54 | A102 | A104 | A152 | A153 | A154 | A202 | A203 | A204 | A252 | A253 | A254 | A302 | A304 | A353
equation "\"d4\" = Length"
equation "\"d10\" = d9"
equation "\"d11\" = d9"
equation "\"d12\" = 0.5 * Length"
equation "\"d14\" = d13"
equation "\"d41\" = d9"
equation "\"d68\" = d60"
equation "\"d71\" = d60"
equation "\"Length\" = 750"
body "Solid1"
